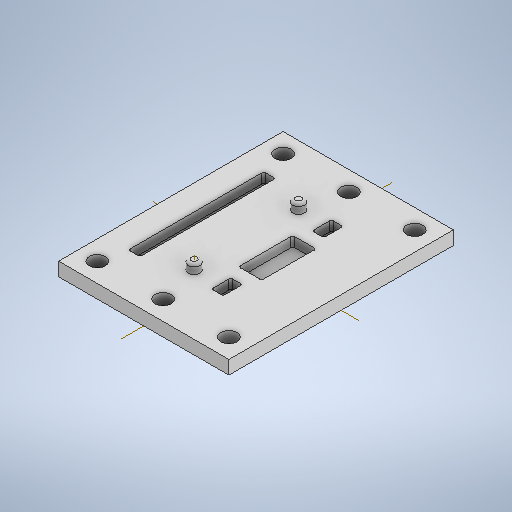
# Autodesk Inventor part: connector-houseing-bottom-plate
Saved by Autodesk Inventor 2025 (Build 290162000, 162)
## iProperties
Created: 2025-05-30
Part Number: connector-houseing-bottom-plate
Material: Generic
Document SubType Name: Modeling
Designer: mumin
Density: 1 g/cm^3
Appearance: Default
Author: mumin
Autodesk Inventor part; units mm, degrees
ref_plane "YZ Plane" through (0, 0, 0) normal (1, 0, 0) x (0, 1, 0)
ref_plane "XZ Plane" through (0, 0, 0) normal (0, 1, 0) x (-1, 0, 0)
ref_plane "XY Plane" through (0, 0, 0) normal (0, 0, 1) x (1, 0, 0)
sketch "Sketch1" plane through (0, 0, 0) normal (0, 1, 0) x (-1, 0, 0)
  line L0 (22, 29) -> (-22, 29)
  line L1 (-22, 29) -> (-22, -29)
  line L2 (-22, -29) -> (22, -29)
  line L3 (22, -29) -> (22, 29)
  point P0 (0, 0)
  point P1 (0, -29)
  dimension "d2" = 44
  dimension "d3" = 58
  constraints: 8 end point, 2 parallel, 1 horizontal, 1 midpoint, 1 perpendicular
  measures "d2" distance of L2.end L1.end
  measures "d3" distance of L1.end L0.end
extrude "Extrusion1" add sketch "Sketch1" along normal blind 3.5
sketch "Sketch2" plane through (0, 3.5, 0) normal (0, 1, 0) x (1, 0, 0)
  line L0 (0, 40.6) -> (0, -40.6) projected
  line L1 (22, 29) -> (-22, 29) projected
  point P0 (0, 0)
  point P1 (0, 24)
  dimension "d22" = 5
  constraints: 1 point on line
  measures "d22" distance from line of L1 point (0, 24)
hole "Hole1" at (0, 3.5, -24) direction (0, -1, 0) diameter 4.2 end through all
pattern_linear "Rectangular Pattern1" count 2 spacing 17 along (-1, 0, 0) count 2 spacing 17 along (1, 0, 0) of "Hole1"
mirror "Mirror1" about plane through (0, 0, 0) normal (0, 0, 1) of "Hole1", "Rectangular Pattern1"
sketch "Sketch3" plane through (0, 3.5, 0) normal (0, 1, 0) x (1, 0, 0)
  circle A0 centre (-2.5, 13.5) radius 1.5
  line L0 (0, 40.6) -> (0, -40.6) projected
  line L1 (-30.8, 0) -> (30.8, 0) projected
  circle A1 centre (-2.5, -13.5) radius 1.5
  point P0 (0, 0)
  dimension "d29" = 3
  dimension "d30" = 2.5
  dimension "d31" = 13.5
  constraints: 2 centre point, 1 symmetric about line, 1 other
  measures "d29" diameter of A0
  measures "d30" distance from line of L0 A0.centre
  measures "d31" distance from line of L1 A0.centre
extrude "Extrusion2" add sketch "Sketch3" along normal blind 2.5
fillet "Fillet1" radius 0.75 2 edges at (-4, 6, -13.5) (-4, 6, 13.5)
sketch "Sketch4" plane through (0, 0, 0) normal (0, 0, 1) x (1, 0, 0)
  line L0 (-15.5, 3.5) -> (-12.5, 3.5)
  line L1 (-12.5, 3.5) -> (-12.5, 1)
  line L2 (-12.5, 1) -> (-15.5, 1)
  line L3 (-15.5, 1) -> (-15.5, 3.5)
  line L4 (-22, 3.5) -> (22, 3.5) projected
  point P0 (0, 0)
  point P1 (0, 3.5)
  point P2 (-14, 3.5)
  dimension "d35" = 2.5
  dimension "d36" = 3
  dimension "d39" = 14
  constraints: 8 end point, 2 midpoint, 2 parallel, 1 collinear, 1 horizontal, 1 perpendicular
  measures "d35" distance of L0.end L1.end
  measures "d36" distance of L1.end L2.end
  measures "d39" distance of point (0, 3.5) point (-14, 3.5)
extrude "Extrusion3" cut sketch "Sketch4" along normal mid plane 35
sketch "Sketch5" plane through (0, 0, 0) normal (0, 0, 1) x (1, 0, 0)
  line L0 (2.5, 3.5) -> (8.5, 3.5)
  line L1 (8.5, 3.5) -> (8.5, 1)
  line L2 (8.5, 1) -> (2.5, 1)
  line L3 (2.5, 1) -> (2.5, 3.5)
  line L4 (-22, 3.5) -> (22, 3.5) projected
  line L5 (-2.5, 7.2) -> (-2.5, -1.2) projected
  point P0 (0, 0)
  point P1 (5.5, 3.5)
  dimension "d40" = 6
  dimension "d41" = 2.5
  dimension "d42" = 8
  constraints: 8 end point, 2 parallel, 1 collinear, 1 horizontal, 1 midpoint, 1 perpendicular
  measures "d40" distance of L1.end L2.end
  measures "d41" distance of L0.end L1.end
  measures "d42" distance from line of L5 point (5.5, 3.5)
extrude "Extrusion4" cut sketch "Sketch5" along normal mid plane 14
sketch "Sketch6" plane through (0, 3.5, 0) normal (0, 1, 0) x (1, 0, 0)
  line L0 (7, -10.5) -> (4, -10.5)
  line L1 (4, -10.5) -> (4, -15.5)
  line L2 (4, -15.5) -> (7, -15.5)
  line L3 (7, -15.5) -> (7, -10.5)
  line L4 (8.5, 7) -> (8.5, -7) projected
  line L5 (8.5, -7) -> (2.5, -7) projected
  point P0 (0, 0)
  point P1 (5.5, -10.5)
  dimension "d45" = 3
  dimension "d46" = 5
  dimension "d47" = 3
  dimension "d48" = 3.5
  constraints: 8 end point, 2 parallel, 1 horizontal, 1 midpoint, 1 perpendicular
  measures "d45" distance of L2.end L1.end
  measures "d46" distance of L1.end L0.end
  measures "d47" distance from line of L4 point (5.5, -10.5)
  measures "d48" distance between parallel lines of L0 L5
extrude "Extrusion5" cut sketch "Sketch6" against normal blind 2.5
mirror "Mirror2" about plane through (0, 0, 0) normal (0, 0, 1) of "Extrusion5"
fillet "Fillet2" radius 0.5 16 edges at (-15.5, 2.25, -17.5) (-12.5, 2.25, -17.5) (-15.5, 2.25, 17.5) (-12.5, 2.25, 17.5) (2.5, 2.25, 7) (8.5, 2.25, 7) (7, 2.25, 15.5) (7, 2.25, -10.5) (7, 2.25, 10.5) (8.5, 2.25, -7) (7, 2.25, -15.5) (2.5, 2.25, -7) (4, 2.25, -15.5) (4, 2.25, -10.5) (4, 2.25, 15.5) (4, 2.25, 10.5)
body "Solid1"
